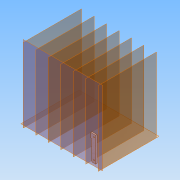
# Autodesk Inventor part: Selection_Ramp 1_Mid piece
Saved by Autodesk Inventor 2018.1 (Build 221171000, 171)
## iProperties
Created: 2019-02-07
Part Number: Selection_Ramp 1_Mid piece
Material: Wood (Cherry)
Document SubType Name: Modeling
Designer: James
Density: 0.63 g/cm^3
Appearance: Cherry - Natural Low Gloss
Author: James
Autodesk Inventor part; units mm, degrees
ref_plane "YZ Plane" through (0, 0, 0) normal (1, 0, 0) x (0, 1, 0)
ref_plane "XZ Plane" through (0, 0, 0) normal (0, 1, 0) x (-1, 0, 0)
ref_plane "XY Plane" through (0, 0, 0) normal (0, 0, 1) x (1, 0, 0)
derived "Selection_Skeleton.ipt"
ref_plane "Ground" through (0, 0, 0) normal (0, 1, 0) x (-1, 0, 0)
ref_plane "LHS inner" through (0, 0, 0) normal (1, 0, 0) x (0, 1, 0)
ref_plane "RHS inner" through (300, 0, 0) normal (1, 0, 0) x (0, 1, 0)
ref_plane "Lane 1" through (50, 0, 0) normal (1, 0, 0) x (0, 1, 0)
ref_plane "Lane 2" through (100, 0, 0) normal (1, 0, 0) x (0, 1, 0)
ref_plane "Lane 3" through (150, 0, 0) normal (1, 0, 0) x (0, 1, 0)
ref_plane "Lane 4" through (200, 0, 0) normal (1, 0, 0) x (0, 1, 0)
ref_plane "Lane 5" through (250, 0, 0) normal (1, 0, 0) x (0, 1, 0)
ref_plane "Back" through (0, 0, 0) normal (0, 0, 1) x (1, 0, 0)
sketch "Sketch1" plane through (0, 0, 0) normal (0, 1, 0) x (-1, 0, 0)
  line L0 (-280, 100) -> (-280, 0)
  line L1 (-280, 0) -> (-265, 0)
  line L2 (-50, -20) -> (-50, 120) projected
  line L3 (-100, -20) -> (-100, 120) projected
  line L4 (-336, 0) -> (56, 0) projected
  line L5 (-250, -20) -> (-250, 120) projected
  line L6 (-265, 0) -> (-260, 100)
  line L7 (-280, 100) -> (-260, 100)
  point P0 (0, 0)
  dimension "d23" = 15
  dimension "d24" = 15
  dimension "d25" = 100
  dimension "d26" = 5
  constraints: 8 end point, 1 collinear, 1 horizontal, 1 vertical
  measures "d23" distance of L0.end L1.end
  measures "d24" distance from line of L1.end L5
  measures "d25" distance of L0.start L0.end
  measures "d26" horizontal distance of L1.end L6.end
extrude "Extrusion1" add sketch "Sketch1" along normal blind 5
sketch "Sketch2" plane through (0, 5, 0) normal (0, 1, 0) x (1, 0, 0)
  line L0 (280, 0) -> (265, 0) projected
  line L1 (260, -100) -> (280, -100) projected
  point P0 (0, 0)
  point P1 (272.5, -10)
  point P2 (272.5, -90)
  dimension "d10" = 10
  dimension "d11" = 80
  dimension "d12" = 7.5
  dimension "d13" = 7.5
  dimension "d27" = 10
  constraints: 1 vertical alignment
  measures "d10" distance from line of point (272.5, -10) L0
  measures "d11" distance of point (272.5, -90) point (272.5, -10)
  measures "d12" horizontal distance of point (272.5, -10) L0.start
  measures "d13" horizontal distance of point (272.5, -10) L0.end
  measures "d27" distance from line of point (272.5, -90) L1
hole "Hole1" at (272.5, 5, 10) at (272.5, 5, 90) direction (0, -1, 0) diameter 4.5 end through all countersink diameter 9.4 countersink angle 90 clearance for "Flat Head Machine Screw" size "M4" standard "Ansi Metric M Profile"
equation "\"d10\" = d27"
equation "\"d12\" = d13"
body "Solid1"
